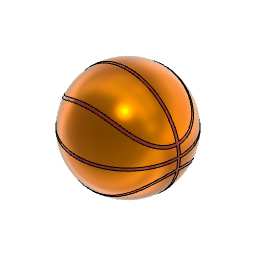
basket ball v1 (Autodesk Fusion 360 design; units mm, degrees)
Autodesk Fusion 360 part; units mm, degrees
sketch "Sketch1" plane through (0, 0, 0) normal (1, 0, 0) x (0, 1, 0)
  line L0 (0, 0) -> (0, 40.2409) construction
  line L1 (-2.5, 94.9997) -> (2.5, 95.0072)
  line L2 (-2.5, 2.5) -> (-95.0072, 2.5)
  line L3 (-2.5, 0) -> (-40.2409, 0) construction
  line L4 (-2.5, -2.5) -> (-2.5, -95.0072)
  line L5 (0, -2.5) -> (0, -40.2409) construction
  line L6 (2.5, -2.5) -> (95.0072, -2.5)
  line L7 (2.5, 0) -> (40.2409, 0) construction
  line L8 (-0.0003, 2.5) -> (0, 2.5)
  line L9 (2.5, 2.5) -> (94.9997, 2.5)
  line L10 (0.0003, -2.5) -> (0, -2.5)
  line L11 (-2.5, -2.5) -> (-94.9997, -2.5)
  line L12 (-2.5, -0.0003) -> (-2.5, 0)
  line L13 (-2.5, 2.5) -> (-2.5, 94.9997)
  line L14 (2.5, 0.0003) -> (2.5, 0)
  line L15 (2.5, -2.5) -> (2.5, -94.9997)
  line L16 (94.9997, 2.5) -> (95.0072, -2.5)
  line L17 (2.5, -94.9997) -> (-2.5, -95.0072)
  line L18 (-94.9997, -2.5) -> (-95.0072, 2.5)
  arc A0 (2.5, 23.5529) -> (-2.5, 23.5349) centre (-0.2584, 95.5) ccw
  line L19 (2.5, 2.5) -> (2.5, 18.5494)
  line L20 (2.5, 23.5529) -> (2.5, 95.0072)
  arc A1 (2.5, 18.5494) -> (-2.5, 18.5326) centre (-0.2584, 95.5) ccw
  arc A2 (-2.5, -23.5349) -> (2.5, -23.5529) centre (-0.2584, -95.5) ccw
  arc A3 (-2.5, -18.5326) -> (2.5, -18.5494) centre (-0.2584, -95.5) ccw
  dimension "d1" = 95
  dimension "d4" = 2.5
  dimension "d7" = 154
  dimension "d8" = 93
  constraint coincident L0.start origin
  constraint vertical L0
  constraint vertical L19
  constraint vertical L12
  constraint coincident L2.start L12
  constraint coincident L0 L8.end
  constraint collinear L8 L9
  constraint collinear L10 L11
  constraint coincident L6.start L14
  constraint collinear L12 L13
  constraint collinear L14 L15
  constraint parallel L16 L18
  constraint symmetric L7 A1 A3
  constraint symmetric L7 A0 A2
  constraint concentric A0 A1
  constraint coincident L13 A0.end
  constraint coincident A0.start L19
  constraint collinear L19 L20
  constraint coincident L13 A1.end
  constraint coincident L4 A2.start
  constraint coincident L15 A2.end
  constraint coincident L15 A3.end
  constraint coincident L4 A3.start
  measures "d1" distance of L12.start L1.start
  measures "d4" horizontal distance of L0.start L12.start
  measures "d7" diameter of A1
  measures "d8" vertical distance of L9.end A0.centre
sphere "SpherePrimitive1" add diameter 190 placed x (0, 1, 0) y (0, 0, 1) z (1, 0, 0) at (0, 0, 0) makes body 1
extrude "Extrude1" cut sketch "Sketch1" along normal mid plane 732.056 contours L2 L4 L6 L9 L11 L13 L15 L16 L17 L18 L19 A1 | L4 L15 A2 A3 bodies 1 makes body 2 at (-28.2259, 45.5678, -2.5) makes body 3 at (-28.2259, -45.5678, -2.5) makes body 4 at (-28.2259, -45.5678, 2.5) makes body 5 at (-28.2259, 45.5678, 2.5) makes body 6 at (38.4906, 17.1795, -85.1372) makes body 7 at (38.496, -17.2749, -85.1154) makes body 8 at (38.4906, 17.1795, 85.1372)
sphere "SpherePrimitive2" add diameter 189.4 placed x (1, 0, 0) y (0, 1, 0) z (0, 0, 1) at (0, 0, 0) separate body makes body 9
